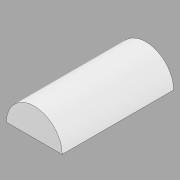
# Autodesk Inventor part: Greenhouse_no_holes
Saved by Autodesk Inventor 2022 (Build 260153000, 153)
## iProperties
Created: 2021-09-02
Part Number: Greenhouse_no_holes
Material: Generic
Document SubType Name: Modeling
Designer: Ben
Density: 1 g/cm^3
Appearance: Smooth - White
Author: Ben
## iProperties of the stored document Greenhouse_3DPrint.ipt
Created: 2021-09-02
Part Number: Greenhouse_3DPrint
Material: Generic
Document SubType Name: Modeling
Designer: Ben
Density: 1 g/cm^3
Appearance: Default
Author: Ben
Autodesk Inventor part; units mm, degrees
ref_plane "YZ Plane" through (0, 0, 0) normal (1, 0, 0) x (0, 1, 0)
ref_plane "XZ Plane" through (0, 0, 0) normal (0, 1, 0) x (-1, 0, 0)
ref_plane "XY Plane" through (0, 0, 0) normal (0, 0, 1) x (1, 0, 0)
sketch "Sketch1" plane through (0, 0, 0) normal (0, 0, 1) x (1, 0, 0)
  arc A0 (31.75, 0) -> (-31.75, 0) centre (0, 0) ccw
  line L0 (-31.75, 0) -> (31.75, 0)
  dimension "diameter" = 63.5
  constraints: 2 end point, 2 point on circle, 1 centre point, 1 coincident, 1 horizontal
  measures "diameter" diameter of A0
extrude "Extrusion1" add sketch "Sketch1" along normal blind 127
equation "\"width\" = 2 * diameter"
body "Solid1"
